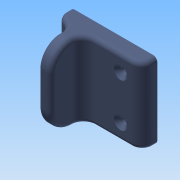
# Autodesk Inventor part: магнитный  держатель
Saved by Autodesk Inventor 2017 (Build 210142000, 142)
## iProperties
Part Number: магнитный  держатель
Material: Типовые
Document SubType Name: Modeling
Designer: chucha
Density: 1 g/cm^3
Appearance: Резина — синяя
Mass: 11.6021 g
Surface Area: 48.479 cm^2
Volume: 11.6021 cm^3
Author: chucha
Autodesk Inventor part; units mm, degrees
ref_plane "YZ Plane" through (0, 0, 0) normal (1, 0, 0) x (0, 1, 0)
ref_plane "XZ Plane" through (0, 0, 0) normal (0, 1, 0) x (-1, 0, 0)
ref_plane "XY Plane" through (0, 0, 0) normal (0, 0, 1) x (1, 0, 0)
sketch "Эскиз1" plane through (0, 0, 0) normal (0, 1, 0) x (-1, 0, 0)
  line L0 (-20, -17.5) -> (20, -17.5)
  line L1 (20, -17.5) -> (20, 17.5)
  line L2 (20, 17.5) -> (-20, 17.5)
  line L3 (-20, 17.5) -> (-20, -17.5)
  line L4 (-20, -17.5) -> (20, 17.5) construction
  line L5 (20, -17.5) -> (-20, 17.5) construction
  line L6 (-10, 17.5) -> (-10, -17.5) construction
  circle A0 centre (-10, 10) radius 1.5
  circle A1 centre (-10, -10) radius 1.5
  line L7 (0, 0) -> (-17.0059, 0) construction
  line L8 (5.5, -10.25) -> (16, -10.25)
  line L9 (16, -10.25) -> (16, 10.25)
  line L10 (16, 10.25) -> (5.5, 10.25)
  line L11 (5.5, 10.25) -> (5.5, -10.25)
  line L12 (5.5, -10.25) -> (16, 10.25) construction
  line L13 (16, -10.25) -> (5.5, 10.25) construction
  circle A2 centre (10.75, 0) radius 1.5
  point P0 (10.75, 0)
  point P1 (10.75, 0)
  dimension "d0" = 3
  dimension "d1" = 3
  dimension "d2" = 20
  dimension "d3" = 10
  dimension "d4" = 35
  dimension "d5" = 10.5
  dimension "d6" = 20.5
  dimension "d14" = 3
  dimension "d17" = 4
  dimension "d18" = 20
  constraints: 28 end point, 5 midpoint, 5 point on line, 4 parallel, 3 centre point, 3 horizontal, 3 perpendicular, 1 coincident, 1 symmetric about line
  measures "d0" diameter of A0
  measures "d1" diameter of A1
  measures "d2" distance of A1.centre A0.centre
  measures "d3" distance between parallel lines of L3 L6
  measures "d4" distance between parallel lines of L0 L2
  measures "d5" distance between parallel lines of L11 L9
  measures "d6" distance between parallel lines of L8 L10
  measures "d14" diameter of A2
  measures "d17" distance between parallel lines of L1 L9
  measures "d18" distance from line of L7.start L3
extrude "Выдавливание1" add sketch "Эскиз1" along normal blind 7 contours L3 L2 L1 L0
extrude "Выдавливание2" add sketch "Эскиз1" along normal blind 3.8 contours L11 L10 L9 L8 | A2
chamfer "Фаска1" distance 1.5 angle 45 2 edges at (11.5, 0, -10) (11.5, 0, 10)
extrude "Выдавливание3" add sketch "Эскиз1" along normal blind 6 contours A2
fillet "Сопряжение1" radius 5 1 edges at (20, 0, 0)
fillet "Сопряжение2" radius 5 1 edges at (-20, 0, 0)
sketch "Эскиз3" plane through (0, 0, 0) normal (0, -1, 0) x (1, 0, 0)
  line L0 (-15, 17.5) -> (15, 17.5) projected
  line L1 (-7, -17.5) -> (-13, -17.5)
  line L2 (-13, -17.5) -> (-13, 17.5)
  line L3 (-13, 17.5) -> (-7, 17.5)
  line L4 (-7, 17.5) -> (-7, -17.5)
  line L5 (-7, -17.5) -> (-13, 17.5) construction
  line L6 (-13, -17.5) -> (-7, 17.5) construction
  point P0 (0, 0)
  point P1 (-10, 0)
  dimension "d27" = 6
  dimension "d28" = 10
  constraints: 12 end point, 2 midpoint, 2 parallel, 1 horizontal, 1 perpendicular, 1 point on line
  measures "d27" distance between parallel lines of L2 L4
  measures "d28" distance of point (0, 0) point (-10, 0)
extrude "Выдавливание5" add sketch "Эскиз3" along normal blind 15
fillet "Сопряжение4" radius 10 2 edges at (-10, -15, 17.5) (-10, -15, -17.5)
fillet "Сопряжение5" radius 5 2 edges at (-13, 0, 0) (-7, 0, 0)
fillet "Сопряжение6" radius 2 22 edges at (-13, -15, 0) (-13, -12.0711, -14.5711) (-13, -4.7697, -17.5) (-13.9689, -1.5814, -17.5) (-19.0311, 2.042, -17.5) (-20, 6, -17.5) (-13, -4.7697, 17.5) (-13.9689, -1.5814, 17.5) (-19.0311, 2.042, 17.5) (-20, 6, 17.5) (-13, -12.0711, 14.5711) (-5.5355, -1.4645, 17.5) (6.5, 0, 17.5) (18.5355, 1.4645, 17.5) (20, 6, 17.5) (-7, -15, 0) (-7, -12.0711, -14.5711) (-5.5355, -1.4645, -17.5) (6.5, 0, -17.5) (18.5355, 1.4645, -17.5) (20, 6, -17.5) (-7, -12.0711, 14.5711)
sketch "Эскиз4" plane through (-10.75, 6, 0) normal (0, 1, 0) x (1, 0, 0)
  circle A0 centre (0, 0) radius 1.5 projected
  point P0 (10.75, 0)
extrude "Выдавливание6" cut sketch "Эскиз4" against normal blind 10
